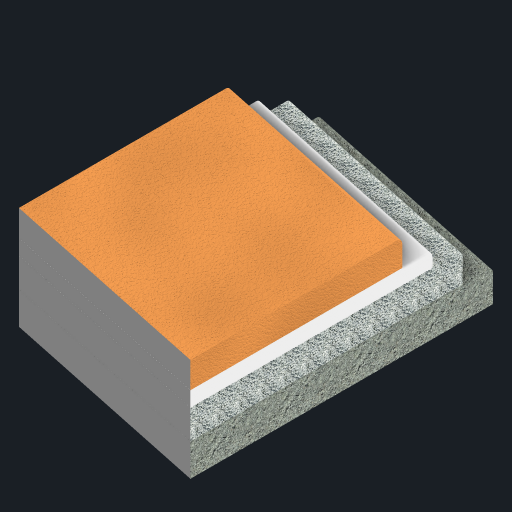
# Autodesk Inventor part: 부품1
Saved by Autodesk Inventor 2024.1 (Build 281209000, 209)
## iProperties
Created: 2024-01-19
Part Number: 부품1
Material: 일반
Document SubType Name: Modeling
Designer: KBU
Density: 1 g/cm^3
Appearance: 기본값
Author: KBU
Autodesk Inventor part; units mm, degrees
ref_plane "YZ Plane" through (0, 0, 0) normal (1, 0, 0) x (0, 1, 0)
ref_plane "XZ Plane" through (0, 0, 0) normal (0, 1, 0) x (-1, 0, 0)
ref_plane "XY Plane" through (0, 0, 0) normal (0, 0, 1) x (1, 0, 0)
sketch "스케치8" plane through (0, 0, 0) normal (0, 0, 1) x (1, 0, 0)
  line L0 (0, 0) -> (0, 160)
  line L1 (0, 160) -> (-850, 387.7568)
  line L2 (-850, 387.7568) -> (-850, 227.7568)
  line L3 (-850, 227.7568) -> (0, 0)
  line L4 (-40.1649, 0) -> (36.8005, 0)
  line L5 (-850, 387.7568) -> (-850, 737.7568)
  line L6 (-850, 737.7568) -> (0, 510)
  line L7 (0, 510) -> (0, 160)
  line L8 (-850, 532.7568) -> (0, 305)
  line L9 (0, 380) -> (-850, 607.7568)
  point P0 (0, 500)
  dimension "d23" = 15
  dimension "d24" = 850
  dimension "d25" = 510
  dimension "d26" = 145
  dimension "d27" = 75
  dimension "d28" = 130
  dimension "d40" = 160
  constraints: 20 end point, 6 parallel, 6 point on line, 2 horizontal, 2 vertical
  measures "d23" angle of L3 L4
  measures "d24" distance between parallel lines of L0 L2
  measures "d25" distance of L2.end L5.end
  measures "d26" distance of L1.end L8.start
  measures "d27" distance of L9.end L8.start
  measures "d28" distance of point (-850, 737.757) L9.end
  measures "d40" distance of L1.end L2.end
extrude "돌출9" add sketch "스케치8" against normal blind 1500 contours L3 L2 L1 L0
extrude "돌출10" add sketch "스케치8" against normal blind 1350 separate body contours L1 L5 L8 L7
extrude "돌출11" add sketch "스케치8" against normal blind 1200 separate body contours L8 L5 L9 L7
extrude "돌출12" add sketch "스케치8" against normal blind 1050 separate body contours L9 L5 L6 L7
fillet "모깎기2" radius 25 4 edges at (-425, 273.8784, -1500) (-425, 418.8784, -1350) (-425, 493.8784, -1200) (-425, 623.8784, -1050)
